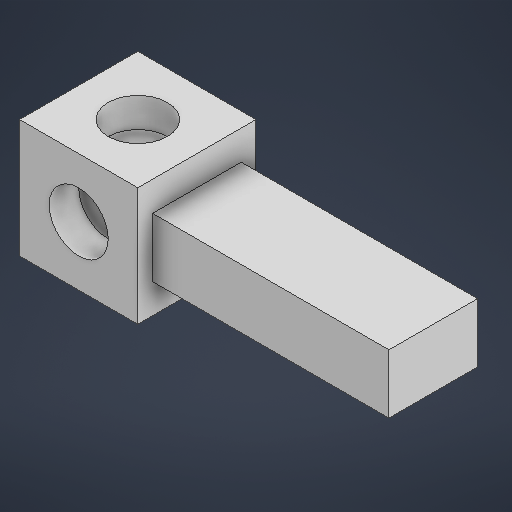
# Autodesk Inventor part: calibration_tool
Saved by Autodesk Inventor 2026.1 (Build 301233020, 233B)
## iProperties
Created: 2025-11-09
Part Number: calibration_tool
Material: Generic
Document SubType Name: Modeling
Designer: Piotrek
Density: 1 g/cm^3
Appearance: Default
Author: Piotrek
Autodesk Inventor part; units mm, degrees
ref_plane "YZ Plane" through (0, 0, 0) normal (1, 0, 0) x (0, 1, 0)
ref_plane "XZ Plane" through (0, 0, 0) normal (0, 1, 0) x (-1, 0, 0)
ref_plane "XY Plane" through (0, 0, 0) normal (0, 0, 1) x (1, 0, 0)
sketch "Sketch1" plane through (0, 0, 0) normal (0, 1, 0) x (-1, 0, 0)
  line L0 (-20, 7.5) -> (20, 7.5)
  line L1 (20, 7.5) -> (20, -7.5)
  line L2 (20, -7.5) -> (-20, -7.5)
  line L3 (-20, -7.5) -> (-20, 7.5)
  line L4 (-20, 7.5) -> (20, -7.5) construction
  line L5 (20, 7.5) -> (-20, -7.5) construction
  line L6 (20, 7.5) -> (40, 7.5)
  line L7 (40, 7.5) -> (40, -7.5)
  line L8 (40, -7.5) -> (20, -7.5)
  line L9 (20, -7.5) -> (20, 7.5)
  line L10 (20, 10) -> (40, 10)
  line L11 (40, 10) -> (40, -10)
  line L12 (40, -10) -> (20, -10)
  line L13 (20, -10) -> (20, 10)
  line L14 (20, 10) -> (40, -10) construction
  line L15 (40, 10) -> (20, -10) construction
  point P0 (0, 0)
  point P1 (30, 0)
  point P2 (20, -7.5)
  point P3 (40, -7.5)
  point P4 (20, 7.5)
  dimension "d0" = 40
  dimension "d1" = 15
  dimension "d2" = 20
  dimension "d3" = 20
  dimension "d4" = 20
  constraints: 32 end point, 6 parallel, 4 midpoint, 3 horizontal, 3 perpendicular, 2 collinear
  measures "d0" distance of L1.end L2.end
  measures "d1" distance of L0.end L1.end
  measures "d2" distance of L7.end L8.end
  measures "d3" distance of L11.end L12.end
  measures "d4" distance of L10.end L11.end
extrude "Extrusion1" add sketch "Sketch1" along normal mid plane 10 contours L0 L1 L2 L3 | L6 L7 L8 L1
extrude "Extrusion2" add sketch "Sketch1" along normal mid plane 20 contours L6 L7 L8 L1 | L13 L10 L11 L6 | L8 L11 L12 L13
sketch "Sketch3" plane through (-40, -10, 10) normal (-1, 0, 0) x (0, 0, 1)
  circle A0 centre (-10, 10) radius 5
  dimension "d12" = 10
  constraints: 1 centre point, 1 coincident
  measures "d12" diameter of A0
sketch "Sketch4" plane through (-40, 10, 10) normal (0, 0, 1) x (1, 0, 0)
  line L0 (20, 0) -> (20, -20) projected
  line L1 (0, 0) -> (20, 0) projected
  line L2 (0, -20) -> (0, 0) projected
  line L3 (20, -20) -> (0, -20) projected
  circle A0 centre (10, -10) radius 5
  point P0 (40, -10)
  dimension "d13" = 10
  constraints: 1 centre point
  measures "d13" diameter of A0
sketch "Sketch2" plane through (0, 10, 0) normal (0, 1, 0) x (1, 0, 0)
  line L0 (-20, -10) -> (-20, 10) projected
  line L1 (-20, 10) -> (-40, 10) projected
  line L2 (-40, 10) -> (-40, -10) projected
  line L3 (-40, -10) -> (-20, -10) projected
  circle A0 centre (-30, 0) radius 5
  point P0 (0, 0)
  dimension "d9" = 10
  constraints: 1 centre point
  measures "d9" diameter of A0
extrude "Extrusion3" cut sketch "Sketch2" against normal blind 5 contours A0
extrude "Extrusion4" cut sketch "Sketch3" against normal blind 5
extrude "Extrusion5" cut sketch "Sketch4" against normal blind 5 contours A0
sketch "Sketch5" plane through (0, -5, 0) normal (0, -1, 0) x (1, 0, 0)
  line L0 (-20, 7.5) -> (-20, -7.5) projected
  line L1 (-20, -7.5) -> (20, -7.5) projected
  line L2 (20, -7.5) -> (20, 7.5) projected
  line L3 (20, 7.5) -> (-20, 7.5) projected
  line L4 (20, 0) -> (-20, 0)
  circle A0 centre (5, 0) radius 1.5
  point P0 (0, 0)
  dimension "d18" = 3
  dimension "d19" = 15
  constraints: 2 end point, 2 midpoint, 1 centre point, 1 point on line
  measures "d18" diameter of A0
  measures "d19" distance from line of L2 A0.centre
extrude "Extrusion6" cut sketch "Sketch5" against normal blind 5 contours A0 L4 | L4 A0
body "Solid1"
